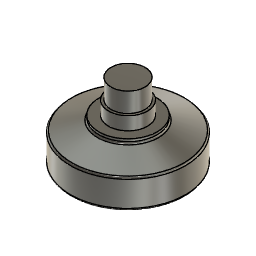
U13 Motor v4 (Autodesk Fusion 360 design; units mm, degrees)
Autodesk Fusion 360 part; units mm, degrees
note: some values were not read from the file. Chosen so that the rebuilt part matches the saved one: which face or edge a step refers to; which pieces of a blend or face edit are solid.
sketch "Sketch1" plane through (0, 0, 0) normal (0, 0, 1) x (1, 0, 0)
  circle A0 centre (0, 0) radius 59.2
  dimension "d1" = 118.4
  constraint coincident A0.centre origin
  measures "d1" diameter of A0
extrude "Extrude1" add sketch "Sketch1" along normal blind 56.8 makes body 1
sketch "Sketch2" plane through (0, 0, 56.8) normal (0, 0, 1) x (-1, 0, 0)
  circle A0 centre (0, 0) radius 59.2
  circle A1 centre (0, 0) radius 30
  dimension "d4" = 60
  constraint coincident A0.centre A1.centre
  measures "d4" diameter of A1
extrude "Extrude2" cut sketch "Sketch2" against normal blind 4 bodies 1
sketch "Sketch5" plane through (0, 0, 0) normal (0, 0, -1) x (1, 0, 0)
  circle A0 centre (0, 0) radius 59.2
  circle A1 centre (0, 0) radius 30
  dimension "d14" = 60
  constraint concentric A0 A1
  measures "d14" diameter of A1
extrude "Extrude4" cut sketch "Sketch5" against normal blind 4 bodies 1
chamfer "Chamfer1" distance 10 distance2 29.2 1 edges at (-55.1938, 21.4076, 52.8) measured on face at (58.9058, 5.8944, 36.5333) on bodies 1
chamfer "Chamfer2" distance 10 distance2 29.2 1 edges at (-55.1938, -21.4076, 4) measured on face at (59.1264, 2.9509, 16.934) on bodies 1
fillet "Fillet1" radius 2 6 edges at (-59.2, 0, 13.9999) (-59.2, 0, 42.802) (-30.0003, 0, 4) (-30.0058, 0, 52.8) (-30, 0, 4) (30, 0, 52.8) on bodies 1
sketch "Sketch6" plane through (0, 0, 0) normal (0, 0, -1) x (1, 0, 0)
  circle A0 centre (0, 0) radius 30
  circle A1 centre (0, 0) radius 25 construction
  line L0 (0, 0) -> (0, 25) construction
  circle A2 centre (0, 25) radius 3
  circle A3 centre (-25, 0) radius 3
  circle A4 centre (0, -25) radius 3
  circle A5 centre (25, 0) radius 3
  dimension "d19" = 50
  dimension "d20" = 6
  dimension "d22" = 360
  constraint coincident A0.centre A1.centre
  constraint coincident A1 L0.end
  constraint vertical L0
  constraint coincident L0.end A2.centre
  measures "d19" diameter of A1
  measures "d20" diameter of A2
extrude "Extrude5" cut sketch "Sketch6" against normal blind 4 contours A2 | A3 | A4 | A5 bodies 1
sketch "Sketch7" plane through (0, 0, 56.8) normal (0, 0, 1) x (-1, 0, 0)
  circle A0 centre (0, 0) radius 30
  circle A1 centre (0, 0) radius 20
  dimension "d25" = 40
  constraint coincident A0.centre A1.centre
  measures "d25" diameter of A1
extrude "Extrude6" add sketch "Sketch7" along normal blind 13.5 contours A1 bodies 1
sketch "Sketch11" plane through (0, 0, 70.3) normal (0, 0, 1) x (-1, 0, 0)
  circle A0 centre (0, 0) radius 20
  circle A1 centre (0, 0) radius 5
  dimension "d38" = 10
  constraint coincident A0.centre A1.centre
  measures "d38" diameter of A1
extrude "Extrude8" add sketch "Sketch11" along normal blind 10.5 from surface at 0.2 separate body contours A1 makes body 2
sketch "Sketch12" plane through (0, 0, 70.3) normal (0, 0, 1) x (-1, 0, 0)
  circle A0 centre (0, 0) radius 20
  circle A1 centre (0, 0) radius 17.5
  dimension "d42" = 35
  constraint concentric A0 A1
  measures "d42" diameter of A1
extrude "Extrude9" add sketch "Sketch12" along normal blind 20 from surface at 0.2 contours A1 bodies 2
copy_body "Body->Comp1" bodies 1 removing the originals makes body 3 in component "U13"
component "U13" placed x (1, 0, 0) y (0, 1, 0) z (0, 0, 1) at (0, 0, 0)
named bodies: "U13"
